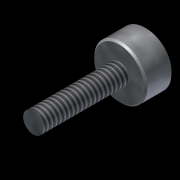
# Autodesk Inventor part: M1.6_5mm
Saved by Autodesk Inventor 2011 (Build 150239000, 239)
## iProperties
Created: 2013-02-08
Part Number: M1.6_5mm
Document SubType Name: Modeling
Designer: arihon
Density: 1 g/cm^3
Author: arihon
Autodesk Inventor part; units mm, degrees
ref_plane "YZ Plane" through (0, 0, 0) normal (1, 0, 0) x (0, 1, 0)
ref_plane "XZ Plane" through (0, 0, 0) normal (0, 1, 0) x (-1, 0, 0)
ref_plane "XY Plane" through (0, 0, 0) normal (0, 0, 1) x (1, 0, 0)
sketch "スケッチ1" plane through (0, 0, 0) normal (0, 0, 1) x (1, 0, 0)
  line L0 (-1.75, 5) -> (-0.2, 5)
  line L1 (1.75, 5) -> (1.75, 3.4)
  line L2 (1.75, 3.4) -> (-1.75, 3.4)
  line L3 (-1.75, 3.4) -> (-1.75, 5)
  line L4 (-0.8, 3.4) -> (-0.2, 3.4)
  line L5 (0.8, 3.4) -> (0.8, -1.6)
  line L6 (0.8, -1.6) -> (-0.2, -1.6)
  line L7 (-0.8, -1.6) -> (-0.8, 3.4)
  line L8 (-0.2, 5) -> (-0.2, -1.6)
  line L9 (-0.2, 5) -> (1.75, 5)
  line L10 (-0.2, 3.4) -> (0.8, 3.4)
  line L11 (-0.2, -1.6) -> (-0.8, -1.6)
  point P0 (0, 0)
  dimension "d0" = 1.6
  dimension "d1" = 0.8
  dimension "d2" = 5
  dimension "d3" = 3.5
  dimension "d4" = 1.75
  dimension "d5" = 1.6
  constraints: 24 end point, 9 parallel, 4 horizontal, 4 perpendicular, 2 point on line
  measures "d0" distance of L5.end L7.start
  measures "d1" distance from line of L5 point (0, 0)
  measures "d2" distance of L5.start L5.end
  measures "d3" distance of L0.start L1.start
  measures "d4" distance from line of L3 point (0, 0)
  measures "d5" distance of L1.start L1.end
revolve "回転1" add sketch "スケッチ1" angle 360 about axis through (-0.2, 5, 0) along (0, -1, 0) contours L0 L8 L2 L3 | L8 L11 L7 L2
sketch "スケッチ2" plane through (-0.2, 5, 0) normal (0, 1, 0) x (1, 0, 0)
  line L0 (0, 0.866) -> (0.75, 0.433)
  line L1 (0.75, 0.433) -> (0.75, -0.433)
  line L2 (0.75, -0.433) -> (0, -0.866)
  line L3 (0, -0.866) -> (-0.75, -0.433)
  line L4 (-0.75, -0.433) -> (-0.75, 0.433)
  line L5 (-0.75, 0.433) -> (0, 0.866)
  point P0 (0, 0)
  dimension "d9" = 1.5
  constraints: 12 end point, 13 other
  measures "d9" distance between parallel lines of L3 L0
extrude "押し出し1" cut sketch "スケッチ2" against normal blind 1
chamfer "面取り1" distance 0.1 angle 45 2 edges at (1.35, 5, 0) (1.35, 3.4, 0)
chamfer "面取り2" distance 0.2 angle 45 6 edges at (0.175, 5, 0.6495) (-0.575, 5, 0.6495) (-0.95, 5, 0) (-0.575, 5, -0.6495) (0.175, 5, -0.6495) (0.55, 5, 0)
thread "ねじ2" size "M1.2x0.25" class "6g" standard "ANSI Metric M Profile" full length
equation "\"d1\" = 0.5 * d0"
equation "\"d4\" = 0.5 * d3"
